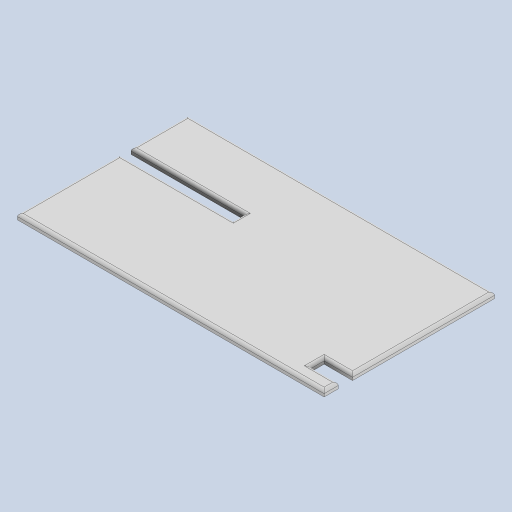
# Autodesk Inventor part: plate
Saved by Autodesk Inventor 2023 (Build 270158000, 158)
## iProperties
Created: 2022-06-10
Part Number: plate
Material: Типовые
Document SubType Name: Modeling
Designer: korra
Density: 1 g/cm^3
Appearance: По умолчанию
Author: korra
Autodesk Inventor part; units mm, degrees
ref_plane "YZ Plane" through (0, 0, 0) normal (1, 0, 0) x (0, 1, 0)
ref_plane "XZ Plane" through (0, 0, 0) normal (0, 1, 0) x (-1, 0, 0)
ref_plane "XY Plane" through (0, 0, 0) normal (0, 0, 1) x (1, 0, 0)
sketch "Эскиз1" plane through (0, 0, 0) normal (0, 1, 0) x (-1, 0, 0)
  line L0 (0, -46.3838) -> (108, -46.3838)
  line L1 (108, 13.6162) -> (0, 13.6162)
  line L2 (108, -46.3838) -> (108, -26.3838)
  line L3 (108, -26.3838) -> (68, -26.3838)
  line L4 (68, -26.3838) -> (68, -22.3838)
  line L5 (68, -22.3838) -> (108, -22.3838)
  line L6 (108, -22.3838) -> (108, 13.6162)
  line L7 (0, 13.6162) -> (0, 8.6162)
  line L8 (0, 8.6162) -> (10, 8.6162)
  line L9 (10, 8.6162) -> (10, 3.6162)
  line L10 (10, 3.6162) -> (0, 3.6162)
  line L11 (0, 3.6162) -> (0, -46.3838)
  point P0 (0, 0)
  dimension "d0" = 108
  dimension "d1" = 60
  dimension "d2" = 20
  dimension "d3" = 40
  dimension "d4" = 4
  dimension "d5" = 5
  dimension "d6" = 10
  dimension "d7" = 5
  constraints: 24 end point, 8 perpendicular, 2 point on line, 2 vertical, 1 horizontal, 1 parallel
  measures "d0" distance of L1.end L1.start
  measures "d1" distance of L1.end L0.start
  measures "d2" distance of L0.end L2.end
  measures "d3" distance of L2.end L3.end
  measures "d4" distance of L3.end L4.end
  measures "d5" distance of L1.end L7.end
  measures "d6" distance of L7.end L8.end
  measures "d7" distance of L8.end L9.end
extrude "Выдавливание1" add sketch "Эскиз1" along normal blind 2
fillet "Сопряжение1" radius 1 12 edges at (-54, 2, 13.6162) (-5, 2, 8.6162) (-10, 2, 6.1162) (-5, 2, 3.6162) (0, 2, -21.3838) (-108, 2, -4.3838) (-88, 2, -22.3838) (-68, 2, -24.3838) (-88, 2, -26.3838) (-108, 2, -36.3838) (-54, 2, -46.3838) (0, 2, 11.1162)
